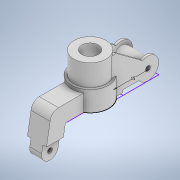
# Autodesk Inventor part: PX9200-16
Saved by Autodesk Inventor 2022.3 (Build 263350000, 350)
## iProperties
Created: 2022-07-15
Part Number: PX9200-16
Material: Generic
Document SubType Name: Modeling
Designer: luis_
Density: 1 g/cm^3
Appearance: Default
Author: luis_
Autodesk Inventor part; units mm, degrees
ref_plane "YZ Plane" through (0, 0, 0) normal (1, 0, 0) x (0, 1, 0)
ref_plane "XZ Plane" through (0, 0, 0) normal (0, 1, 0) x (-1, 0, 0)
ref_plane "XY Plane" through (0, 0, 0) normal (0, 0, 1) x (1, 0, 0)
sketch "Sketch1" plane through (0, 0, 0) normal (0, 1, 0) x (-1, 0, 0)
  line L0 (6, -22.75) -> (-6, -22.75)
  circle A0 centre (0, 0) radius 7.75
  line L1 (6, -7.75) -> (-6, -7.75)
  line L2 (4.0162, 13.75) -> (-3.9838, 13.75)
  line L3 (4.0162, 13.75) -> (4.0162, 7.4875)
  line L4 (6, -4.9054) -> (6, -22.75)
  line L5 (-6, -22.75) -> (-6, -4.9054)
  line L6 (-3.9838, 6.6477) -> (-3.9838, 13.75)
  line L7 (4.0162, 7.4875) -> (4.0162, 6.6282)
  point P0 (0, -7.75)
  dimension "d3" = 15
  constraints: 16 end point, 4 parallel, 4 perpendicular, 4 point on circle, 2 point on line, 1 centre point, 1 coincident, 1 tangent, 1 vertical, 1 other
  measures "d3" distance between parallel lines of L0 L1
extrude "Extrusion1" add sketch "Sketch1" along normal blind 7 contours A0 | L6 L2 L3 L7 A0
extrude "Extrusion2" add sketch "Sketch1" along normal blind 8.4 contours A0
extrude "Extrusion8" add sketch "Sketch1" along normal blind 9 contours L0 L5 L1 L4
sketch "Sketch3" plane through (6, 0, -7.75) normal (1, 0, 0) x (0, 0, -1)
  circle A0 centre (10.5, 4.5) radius 4.5
  line L0 (15, 9) -> (0, 9) projected
  line L1 (15, 0) -> (15, 9) projected
  circle A1 centre (10.5, 4.5) radius 1
  line L2 (15, 0) -> (0, 0) projected
  line L3 (0, 8.4) -> (-15.5, 8.4) projected
  line L4 (0, 8.4) -> (8.255, 8.4)
  line L5 (10.5, 9) -> (0, 9)
  line L6 (0, 9) -> (0, 8.4)
  line L7 (0, 0) -> (0, 8.4) projected
  line L8 (0, 0) -> (10.5, 0)
  line L9 (7.6716, 1) -> (0, 1)
  line L10 (0, 1) -> (0, 0)
  line L11 (0, 0) -> (-12.6554, 0) projected
  line L12 (0, 0) -> (10.5, 0)
  point P0 (-7.75, 0)
  point P1 (10.5, 0)
  point P2 (15, 4.5)
  point P3 (15, 4.5)
  point P4 (0, 1)
  dimension "d25" = 2
  constraints: 14 end point, 4 point on circle, 3 tangent, 2 centre point, 2 horizontal, 2 parallel, 2 point on line, 1 coincident, 1 collinear, 1 midpoint
  measures "d25" diameter of A1
extrude "Extrusion9" cut sketch "Sketch3" against normal blind 20 contours L1 L2 A0 | A0 L0 L1 | A0 L4 L6 L0 | L2 L7 L9 A0 | A1
extrude "Extrusion10" add sketch "Sketch1" along normal blind 8.4 contours L1 A0 L4 | L5 A0 L1
extrude "Extrusion11" cut sketch "Sketch1" along normal blind 1 contours L1 A0 L4 | L5 A0 L1
sketch "Sketch6" plane through (0, 0, 0) normal (1, 0, 0) x (0, 1, 0)
  circle A0 centre (4.5, -18.25) radius 1 projected
  circle A1 centre (4.5, -18.25) radius 3
  arc A2 (2, -14.5083) -> (5.4, -13.8409) centre (4.5, -18.25) ccw
  line L0 (8.4, -16.005) -> (8.4, -4.9054) projected
  line L1 (8.4, -4.9054) -> (1, -4.9054) projected
  line L2 (1, -4.9054) -> (1, -15.4216) projected
  line L3 (1, -4.9054) -> (1, -7.75) projected
  line L4 (1, -7.75) -> (8.4, -7.75)
  line L5 (2, -7.75) -> (2, -14.5083)
  line L6 (5.4, -7.75) -> (5.4, -13.8409)
  circle A3 centre (4.5, -18.25) radius 3
  circle A4 centre (4.5, -18.25) radius 4.5
  line L7 (5.4, -13.8409) -> (5.4, -15.3882)
  line L8 (2, -14.5083) -> (2, -16.5917)
  point P0 (0, 0)
  dimension "d44" = 6
  constraints: 10 end point, 4 centre point, 4 coincident, 4 point on circle, 3 point on line, 2 vertical, 1 parallel, 1 perpendicular, 1 other
  measures "d44" diameter of A3
extrude "Extrusion14" cut sketch "Sketch6" along normal mid plane 10 contours A1 L7 A2 L8
extrude "Extrusion15" cut sketch "Sketch6" along normal mid plane 20 contours L6 L4 L0 A2 | A2 L2 L4 L5
sketch "Sketch7" plane through (0, 8.4, 0) normal (0, 1, 0) x (1, 0, 0)
  circle A0 centre (0, 0) radius 6.75
  dimension "d49" = 13.5
  constraints: 1 centre point, 1 coincident
  measures "d49" diameter of A0
extrude "Extrusion16" add sketch "Sketch7" along normal blind 9
sketch "Sketch8" plane through (0, 17.4, 0) normal (0, 1, 0) x (1, 0, 0)
  circle A0 centre (0, 0) radius 3.5
  dimension "d52" = 7
  constraints: 1 centre point, 1 coincident
  measures "d52" diameter of A0
extrude "Extrusion17" cut sketch "Sketch8" against normal blind 20
sketch "Sketch10" plane through (6, 1, -4.9054) normal (1, 0, 0) x (0, 0, -1)
  line L0 (2.8446, 7.4) -> (0, 7.4) projected
  line L1 (0, 7.4) -> (0, 15.5918)
  line L2 (0, 15.5918) -> (11.0997, 7.4)
  arc A0 (9.603, 1) -> (8.9356, 4.4) centre (13.3446, 3.5) ccw projected
  line L3 (0, 7.4) -> (2.8446, 7.4)
  line L4 (2.8446, 7.4) -> (2.8446, 4.4) projected
  line L5 (2.8446, 4.4) -> (8.9356, 4.4) projected
  line L6 (2.8446, 4.4) -> (8.9356, 4.4)
  arc A1 (11.0997, 7.4) -> (8.9356, 4.4) centre (13.3446, 3.5) ccw
  point P0 (-4.9054, -1)
  constraints: 8 end point, 3 point on circle, 2 collinear, 1 centre point, 1 concentric, 1 vertical
extrude "Extrusion18" add sketch "Sketch10" against normal blind 1
sketch "Sketch11" plane through (0, 17.4, 0) normal (0, 1, 0) x (1, 0, 0)
  line L0 (5, 4.9054) -> (5, 7.75) projected
  line L1 (5, 4.9054) -> (5, 4.5346)
  circle A0 centre (0, 0) radius 6.75 projected
  arc A1 (-6, 4.9054) -> (6, 4.9054) centre (0, 0) ccw projected
  line L2 (6, 4.9054) -> (6, 3.1171)
  arc A2 (6, 3.1171) -> (5, 4.5346) centre (-0.4202, -0.3507) ccw
  line L3 (6, 4.9054) -> (5, 4.9054) projected
  line L4 (6, 4.9054) -> (5, 4.9054)
  line L5 (-6, 4.9054) -> (-6, 3.0923)
  line L6 (-5, 4.5346) -> (-5, 4.9054)
  arc A3 (-5, 4.5346) -> (-6, 3.0923) centre (0, 0) ccw
  line L7 (4.6413, 4.9054) -> (4.6368, 4.9054)
  line L8 (-5, 4.9054) -> (-6, 4.9054)
  point P0 (5.3551, 4.1092)
  constraints: 14 end point, 10 point on circle, 4 perpendicular, 3 collinear, 2 centre point, 2 vertical, 1 concentric
extrude "Extrusion19" add sketch "Sketch11" against normal blind 9 contours L3 L2 A2 L1 | L8 L6 A0 L5
extrude "Extrusion20" cut sketch "Sketch11" against normal blind 0.81 contours L3 L2 A2 L1 | L8 L6 A0 L5
sketch "Sketch12" plane through (-6, 8.4, -4.9054) normal (-1, 0, 0) x (0, 0, 1)
  line L0 (0, 8.19) -> (0, 0) projected
  line L1 (-11.0997, 0) -> (0, 8.1918) projected
  line L2 (0, 8.19) -> (-11.0997, 0)
  line L3 (-2.8446, -3) -> (-10.4828, -3) projected
  arc A0 (-8.9356, -3) -> (-9.603, -6.4) centre (-13.3446, -3.9) ccw projected
  arc A1 (-8.8861, -3) -> (-11.0997, 0) centre (-13.5177, -4.1008) ccw
  line L4 (-8.9356, -3) -> (-2.8446, -3)
  line L5 (-2.8446, 0) -> (-2.8446, -3) projected
  line L6 (-2.8446, 0) -> (0, 0)
  line L7 (0.3708, 0) -> (-2.8446, 0) projected
  point P0 (4.9054, -8.4)
  point P1 (-9.8196, -1.1029)
  constraints: 6 end point, 3 point on circle, 2 collinear, 2 point on line, 1 centre point
extrude "Extrusion21" add sketch "Sketch12" against normal blind 1 contours L0 L6 L5 L3 A1 A0 L1
sketch "Sketch13" plane through (0, 0, 0) normal (0, -1, 0) x (1, 0, 0)
  circle A0 centre (0, 0) radius 4
  circle A1 centre (0, 0) radius 3.5
  dimension "d63" = 8
  constraints: 2 centre point, 2 coincident
  measures "d63" diameter of A0
extrude "Extrusion22" cut sketch "Sketch13" against normal blind 6.75
sketch "Sketch19" plane through (3.9838, 0, 13.75) normal (1, 0, 0) x (0, 0, -1)
  line L0 (0, 0) -> (-7, 0)
  line L1 (-7, 0) -> (-7, 7)
  line L2 (-7, 7) -> (0, 7)
  line L3 (0, 7) -> (0, 0)
  circle A0 centre (-3.5, 3.5) radius 3.5
  point P0 (13.75, 0)
  point P1 (-3.5, 0)
  point P2 (-3.5, 7)
  dimension "d77" = 7
  constraints: 8 end point, 2 parallel, 1 centre point, 1 horizontal, 1 perpendicular
  measures "d77" distance of L1.end L2.end
extrude "Extrusion26" add sketch "Sketch19" against normal blind 8 contours L0 A0 L3 | A0 | A0 L2 L3
sketch "Sketch20" plane through (3.9838, 0, 6.6477) normal (1, 0, 0) x (0, 0, -1)
  arc A0 (-10.6023, 7) -> (-10.6023, 0) centre (-10.6023, 3.5) ccw projected
  line L0 (-10.6023, 3.5) -> (-12.6861, -8.3177) construction
  line L1 (-7.6834, 0) -> (-9.2567, -8.9224)
  line L2 (-16.1155, -7.713) -> (-14.0317, 4.1047)
  arc A1 (-16.1155, -7.713) -> (-9.2567, -8.9224) centre (-12.6861, -8.3177) ccw
  line L3 (-10.6023, 3.5) -> (1.3977, 3.5) construction
  arc A2 (-14.0927, 3.7584) -> (-10.6023, 0) centre (-10.6023, 3.5) ccw
  line L4 (-10.6023, 0) -> (-7.6834, 0)
  line L5 (-10.6023, 0) -> (0, 0) projected
  point P0 (6.6477, 0)
  point P1 (-11.6442, -2.4088)
  dimension "d80" = 12
  dimension "d81" = 100
  constraints: 12 end point, 5 point on circle, 3 tangent, 2 centre point, 2 point on line, 1 concentric, 1 equal length, 1 horizontal, 1 midpoint, 1 parallel
  measures "d80" distance of L0.start L0.end
  measures "d81" angle of L0 L3
extrude "Extrusion27" add sketch "Sketch20" against normal blind 8
sketch "Sketch21" plane through (3.9838, 0, 6.6477) normal (1, 0, 0) x (0, 0, -1)
  arc A0 (-16.1155, -7.713) -> (-9.2567, -8.9224) centre (-12.6861, -8.3177) ccw projected
  circle A1 centre (-12.6861, -8.3177) radius 1
  point P0 (6.6477, 0)
  dimension "d84" = 2
  constraints: 1 centre point, 1 coincident
  measures "d84" diameter of A1
extrude "Extrusion28" cut sketch "Sketch21" against normal blind 8
sketch "Sketch22" plane through (3.9838, 0, 6.6477) normal (1, 0, 0) x (0, 0, -1)
  line L0 (-7.6485, -4.8) -> (-17.7237, -4.8)
  line L1 (-17.7237, -4.8) -> (-17.7237, -18.8)
  line L2 (-17.7237, -18.8) -> (-7.6485, -18.8)
  line L3 (-7.6485, -18.8) -> (-7.6485, -4.8)
  arc A0 (-16.1155, -7.713) -> (-9.2567, -8.9224) centre (-12.6861, -8.3177) ccw projected
  line L4 (-7.6485, -4.8) -> (-17.7237, -18.8) construction
  line L5 (-17.7237, -4.8) -> (-7.6485, -18.8) construction
  line L6 (-17.7237, -4.8) -> (-7.6485, -4.8)
  line L7 (-7.6485, -4.8) -> (-7.6485, -18.8)
  line L8 (-7.6485, -18.8) -> (-17.7237, -18.8)
  line L9 (-17.7237, -18.8) -> (-17.7237, -4.8)
  line L10 (-17.7237, -4.8) -> (-7.6485, -18.8) construction
  line L11 (-7.6485, -4.8) -> (-17.7237, -18.8) construction
  point P0 (6.6477, 0)
  point P1 (-12.6861, -11.8)
  dimension "d87" = 14
  constraints: 24 end point, 4 midpoint, 4 parallel, 2 horizontal, 2 perpendicular, 1 point on circle
  measures "d87" distance of L1.end L0.end
extrude "Extrusion29" cut sketch "Sketch22" against normal blind 1.5
sketch "Sketch23" plane through (-4.0162, 0, 6.6282) normal (-1, 0, 0) x (0, 0, 1)
  line L0 (18.9747, -4.8) -> (6.4365, -4.8)
  line L1 (6.4365, -4.8) -> (6.4365, -18.8)
  line L2 (6.4365, -18.8) -> (18.9747, -18.8)
  line L3 (18.9747, -18.8) -> (18.9747, -4.8)
  arc A0 (9.2762, -8.9224) -> (16.135, -7.713) centre (12.7056, -8.3177) ccw projected
  line L4 (18.9747, -4.8) -> (6.4365, -18.8) construction
  line L5 (6.4365, -4.8) -> (18.9747, -18.8) construction
  point P0 (-6.6282, 0)
  point P1 (12.7056, -11.8)
  dimension "d90" = 14
  constraints: 12 end point, 2 midpoint, 2 parallel, 1 horizontal, 1 perpendicular, 1 point on circle
  measures "d90" distance of L1.end L0.end
extrude "Extrusion30" cut sketch "Sketch23" against normal blind 1.5
body "Solid1"
